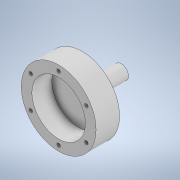
# Autodesk Inventor part: Coupling
Saved by Autodesk Inventor 2020 (Build 240168000, 168)
## iProperties
Created: 2022-06-09
Part Number: Coupling
Material: 일반
Document SubType Name: Modeling
Designer: samsung
Density: 1 g/cm^3
Appearance: 기본값
Author: samsung
Autodesk Inventor part; units mm, degrees
sketch "스케치1" plane through (0, 0, 0) normal (0, 0, 1) x (1, 0, 0)
  line L0 (-2.5, 2.9544) -> (-2.5, 5.4544)
  arc A0 (-2.5, 5.4544) -> (2.5, 5.4544) centre (0, 0) ccw projected
  spline S0 degree 3 poles (-2.5, 5.4544) (-2.4742, 5.4667) (-2.4356, 5.4852) (-2.1794, 5.5919) (-1.9877, 5.6659) (-1.5481, 5.8014) (-1.2695, 5.8724) (-0.6546, 5.9723) (-0.318, 6) (0.318, 6) (0.6546, 5.9723) (1.2695, 5.8724) (1.5481, 5.8014) (1.9877, 5.6659) (2.1794, 5.5919) (2.4356, 5.4852) (2.4742, 5.4667) (2.5, 5.4544) knots 0 0 0 0 0.095508 0.095508 0.191016 0.191016 0.286409 0.286409 0.381802 0.381802 0.477194 0.477194 0.572587 0.572587 0.668095 0.668095 0.763603 0.763603 0.763603 0.763603 projected
  circle A1 centre (0, 0) radius 10
  line L1 (2.5, 5.4544) -> (-2.5, 5.4544)
  line L2 (-2.5, 5.4544) -> (-2.5, 2.9544)
  line L3 (-2.5, 2.9544) -> (2.5, 2.9544)
  line L4 (2.5, 2.9544) -> (2.5, 5.4544)
  line L5 (2.5, 5.4544) -> (-2.5, 5.4544)
  line L6 (-2.5, 5.4544) -> (-2.5, 7.9544)
  line L7 (-2.5, 7.9544) -> (2.5, 7.9544)
  line L8 (2.5, 7.9544) -> (2.5, 5.4544)
  dimension "d0" = 20
  dimension "d87" = 2.5
  dimension "d88" = 2.5
  constraints: 18 end point, 4 parallel, 2 horizontal, 2 perpendicular, 1 centre point, 1 coincident
  measures "d0" diameter of A1
  measures "d87" distance of L0.start L1.end
  measures "d88" distance of L5.end L6.end
ref_plane "작업 평면3" through (0, 0, 0) normal (0, 0, 1) x (1, 0, 0)
sketch "스케치2" plane through (0, 0, 0) normal (0, 0, 1) x (1, 0, 0)
  arc A0 (-2.5, 5.4544) -> (2.5, 5.4544) centre (0, 0) ccw projected
  line L0 (2.5, 8.4544) -> (-2.5, 8.4544) projected
  line L1 (-2.5, 2.4544) -> (-2.5, 8.4544) projected
  line L2 (2.5, 2.4544) -> (2.5, 8.4544) projected
  circle A1 centre (0, 0) radius 16 projected
  circle A2 centre (0, 0) radius 10
  point P0 (0, 0)
  dimension "d19" = 20
  constraints: 1 centre point, 1 coincident
  measures "d19" diameter of A2
extrude "돌출5" add sketch "스케치1" against normal blind 20
ref_plane "작업 평면4" through (0, -10, 0) normal (0, -1, 0) x (1, 0, 0)
extrude "돌출8" add sketch "스케치2" along normal blind 35 contours L1 L0 L2 A0 | A2
sketch "스케치6" plane through (0, 0, 35) normal (0, 0, 1) x (1, 0, 0)
  circle A0 centre (0, 0) radius 52.5
  dimension "d22" = 105
  constraints: 1 centre point, 1 coincident
  measures "d22" diameter of A0
extrude "돌출9" add sketch "스케치6" along normal blind 5
sketch "스케치7" plane through (0, -10, 0) normal (0, -1, 0) x (1, 0, 0)
  line L0 (10, 35) -> (-10, 35) projected
  line L1 (-10, -20) -> (10, -20) projected
  line L2 (-10, 35) -> (-10, -20) projected
  line L3 (10, 35) -> (10, -20) projected
  circle A0 centre (0, -5) radius 3.5
  point P0 (0, 0)
  dimension "d25" = 7
  dimension "d26" = 5
  constraints: 1 centre point
  measures "d25" diameter of A0
  measures "d26" distance of A0.centre point (0, 0)
extrude "돌출10" cut sketch "스케치7" against normal blind 0.46 contours A0
sketch "스케치9" plane through (0, -9.54, 0) normal (0, -1, 0) x (1, 0, 0)
  line L0 (2.9981, -3.194) -> (2.9981, -6.806) projected
  arc A0 (2.9981, -3.194) -> (-2.9981, -3.194) centre (0, -5) ccw projected
  line L1 (-2.9981, -6.806) -> (-2.9981, -3.194) projected
  arc A1 (-2.9981, -6.806) -> (2.9981, -6.806) centre (0, -5) ccw projected
  circle A2 centre (0, -5) radius 1
  point P0 (0, 0)
  dimension "d32" = 2
  constraints: 2 coincident, 1 centre point
  measures "d32" diameter of A2
sketch "스케치10" plane through (0, 0, 40) normal (0, 0, 1) x (1, 0, 0)
  circle A0 centre (0, 0) radius 76
  circle A1 centre (0, 0) radius 10
  circle A2 centre (0, 0) radius 45
  circle A3 centre (0, 0) radius 52.5
  circle A4 centre (0, 0) radius 37.5
  dimension "d35" = 152
  dimension "d36" = 20
  dimension "d62" = 90
  dimension "d71" = 105
  dimension "d72" = 75
  constraints: 5 centre point, 2 coincident
  measures "d35" diameter of A0
  measures "d36" diameter of A1
  measures "d62" diameter of A2
  measures "d71" diameter of A3
  measures "d72" diameter of A4
ref_plane "작업 평면5" through (0, 0, 64) normal (0, 0, 1) x (1, 0, 0)
hole "구멍2" at (0, -9.54, -5) direction (0, 1, 0) diameter 3.242 depth 11.8 tip angle 118 thread size "M4x0.7" class "6H" standard "ISO Metric profile"
extrude "돌출14" add sketch "스케치10" along normal blind 28 contours A2 | A3
sketch "스케치12" plane through (0, 0, 68) normal (0, 0, 1) x (1, 0, 0)
  circle A0 centre (0, 0) radius 45
  point P0 (0, 45)
  point P1 (-38.9711, 22.5)
  point P2 (-38.9711, -22.5)
  point P3 (0, -45)
  point P4 (38.9711, -22.5)
  point P5 (38.9711, 22.5)
  dimension "d75" = 90
  dimension "d78" = 360
  constraints: 1 coincident, 1 vertical alignment, 9 other
hole "구멍3" at (0, 45, 68) at (-38.9711, 22.5, 68) at (-38.9711, -22.5, 68) at (0, -45, 68) at (38.9711, -22.5, 68) at (38.9711, 22.5, 68) direction (0, 0, -1) diameter 4.917 depth 15 tip angle 118 thread size "M6x1" class "6H" standard "ISO Metric profile"
